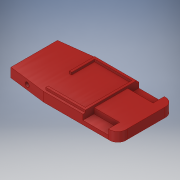
# Autodesk Inventor part: RC_Chassis
Saved by Autodesk Inventor 2019 (Build 230136000, 136)
## iProperties
Created: 2020-12-18
Part Number: RC_Chassis
Material: Generic
Document SubType Name: Modeling
Designer: wahid
Density: 1 g/cm^3
Appearance: Orange-Red
Author: wahid
Autodesk Inventor part; units mm, degrees
ref_plane "YZ Plane" through (0, 0, 0) normal (1, 0, 0) x (0, 1, 0)
sketch "Sketch1" plane through (0, 0, 0) normal (0, 1, 0) x (-1, 0, 0)
  line L0 (304.8, -139.7) -> (203.2, -152.4)
  line L1 (304.8, -12.7) -> (203.2, 0)
  line L2 (304.8, -12.7) -> (304.8, -139.7)
  arc A0 (25.4, 0) -> (0, -25.4) centre (22.225, -22.225) ccw
  line L3 (203.2, 0) -> (25.4, 0)
  arc A1 (0, -127) -> (25.4, -152.4) centre (22.225, -130.175) ccw
  line L4 (203.2, -152.4) -> (25.4, -152.4)
  line L5 (0, -127) -> (0, -25.4)
  point P0 (0, 0)
  point P1 (203.2, -12.7)
  point P2 (203.2, -139.7)
  point P3 (101.6, -12.7)
  point P4 (101.6, -139.7)
  point P5 (101.6, -152.4)
  point P6 (0, -139.7)
  dimension "d8" = 12.7
  dimension "d12" = 101.6
  dimension "d13" = 127
  constraints: 12 end point, 4 point on circle, 2 centre point, 2 horizontal, 1 coincident, 1 perpendicular, 1 vertical
  measures "d8" distance of L1.end point (203.2, -12.7)
  measures "d12" distance of point (101.6, -12.7) point (203.2, -12.7)
  measures "d13" distance of point (101.6, -12.7) point (101.6, -139.7)
extrude "Extrusion1" add sketch "Sketch1" against normal blind 25.4
sketch "Sketch2" plane through (0, 0, 0) normal (0, 1, 0) x (1, 0, 0)
  line L0 (-25.4, 0) -> (-203.2, 0) projected
  line L1 (-203.2, 152.4) -> (-25.4, 152.4) projected
  line L2 (-203.2, 12.7) -> (-101.6, 12.7)
  line L3 (-101.6, 12.7) -> (-101.6, 139.7)
  line L4 (-101.6, 139.7) -> (-203.2, 139.7)
  line L5 (-203.2, 139.7) -> (-203.2, 12.7)
  line L6 (-209.55, 6.35) -> (-95.25, 6.35)
  line L7 (-95.25, 6.35) -> (-95.25, 146.05)
  line L8 (-95.25, 146.05) -> (-209.55, 146.05)
  line L9 (-209.55, 146.05) -> (-209.55, 6.35)
  point P0 (0, 0)
  point P1 (-203.2, 6.35)
  dimension "d23" = 12.7
  dimension "d24" = 101.6
  dimension "d25" = 127
  dimension "d26" = 6.35
  dimension "d27" = 6.35
  dimension "d28" = 114.3
  dimension "d29" = 139.7
  constraints: 16 end point, 4 parallel, 2 horizontal, 2 perpendicular
  measures "d23" distance from line of L0 L2.start
  measures "d24" distance of L4.end L3.end
  measures "d25" distance of L3.end L2.end
  measures "d26" distance from line of L0 point (-203.2, 6.35)
  measures "d27" distance from line of L6.start L5
  measures "d28" distance of L8.end L7.end
  measures "d29" distance of L7.end L6.end
extrude "Extrusion2" add sketch "Sketch2" along normal blind 6.35
ref_plane "Work Plane1" through (-203.2, 0, 0) normal (-0.0012, 0, 1) x (1, 0, 0.0012)
sketch "Sketch7" plane through (-203.2, 0, 0) normal (-0.0012, 0, 1) x (1, 0, 0.0012)
  line L0 (0, 0) -> (0, -25.4) projected
  line L1 (0, -25.4) -> (-101.6158, -25.4) projected
  circle A0 centre (-50.8, -12.7) radius 6.35
  point P0 (203.1998, 0)
  dimension "d41" = 50.8
  dimension "d43" = 12.7
  dimension "d44" = 12.7
  constraints: 1 centre point, 1 coincident
  measures "d41" distance from line of point (-50.8, -12.7) L0
  measures "d43" diameter of A0
  measures "d44" distance from line of L1 A0.centre
extrude "Extrusion4" cut sketch "Sketch7" against normal blind 152.4
ref_plane "Work Plane3" through (-22.225, 0, -152.6256) normal (0, 0, -1) x (-1, 0, 0)
sketch "Sketch11" plane through (0, 0, 0) normal (0, 1, 0) x (1, 0, 0)
  line L0 (-95.25, 0) -> (-25.654, 0)
  line L1 (-25.654, 0) -> (-25.654, 30.48)
  line L2 (-25.654, 30.48) -> (-95.25, 30.48)
  line L3 (-95.25, 30.48) -> (-95.25, 0)
  line L4 (-95.25, 6.35) -> (-95.25, 146.05) projected
  line L5 (-95.25, 152.4) -> (-25.654, 152.4)
  line L6 (-25.654, 152.4) -> (-25.654, 121.92)
  line L7 (-25.654, 121.92) -> (-95.25, 121.92)
  line L8 (-95.25, 121.92) -> (-95.25, 152.4)
  point P0 (0, 0)
  dimension "d59" = 69.596
  dimension "d60" = 30.48
  dimension "d61" = 69.596
  dimension "d62" = 30.48
  constraints: 16 end point, 4 parallel, 2 horizontal, 2 perpendicular
  measures "d59" distance of L2.end L1.end
  measures "d60" distance of L1.end L0.end
  measures "d61" distance of L6.end L7.end
  measures "d62" distance of L5.end L6.end
extrude "Extrusion7" cut sketch "Sketch11" against normal blind 14.732
sketch "Sketch12" plane through (0, 6.35, 0) normal (0, 1, 0) x (1, 0, 0)
  line L0 (-203.2, 22.5806) -> (-203.2, 76.9366)
  line L1 (-203.2, 76.9366) -> (-209.55, 76.9366)
  line L2 (-209.55, 76.9366) -> (-209.55, 22.5806)
  line L3 (-209.55, 76.9366) -> (-203.2, 76.9366)
  line L4 (-203.2, 76.9366) -> (-203.2, 6.35)
  line L5 (-203.2, 6.35) -> (-209.55, 6.35)
  line L6 (-209.55, 6.35) -> (-209.55, 76.9366)
  point P0 (0, 0)
  point P1 (-203.2, 12.7)
  point P2 (-209.55, 6.35)
  point P3 (-209.55, 12.7)
  dimension "d67" = 9.8806
  dimension "d68" = 6.35
  dimension "d69" = 54.356
  constraints: 14 end point, 3 parallel, 1 horizontal, 1 perpendicular
  measures "d67" distance of point (-209.55, 12.7) L2.end
  measures "d68" distance of L1.end L0.end
  measures "d69" distance of L0.end L0.start
extrude "Extrusion9" cut sketch "Sketch12" against normal blind 6.35
body "Solid1"
